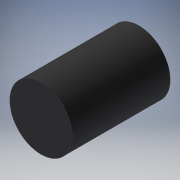
# Autodesk Inventor part: NespressoSpeedfiller-Rod
Saved by Autodesk Inventor 2017 (Build 210142000, 142)
## iProperties
Created: 2018-08-27
Part Number: NespressoSpeedfiller-Rod
Material: Generic
Document SubType Name: Modeling
Designer: 45027374
Density: 1 g/cm^3
Appearance: Default
Author: 45027374
Autodesk Inventor part; units mm, degrees
ref_plane "YZ Plane" through (0, 0, 0) normal (1, 0, 0) x (0, 1, 0)
ref_plane "XZ Plane" through (0, 0, 0) normal (0, 1, 0) x (-1, 0, 0)
ref_plane "XY Plane" through (0, 0, 0) normal (0, 0, 1) x (1, 0, 0)
sketch "Sketch1" plane through (0, 0, 0) normal (0, 1, 0) x (-1, 0, 0)
  line L0 (17.85, 0) -> (-17.85, 0) projected
  line L1 (0, -17.85) -> (0, 17.85) projected
  circle A0 centre (0, 0) radius 12.75
  dimension "d0" = 25.5
  constraints: 1 centre point, 1 coincident
  measures "d0" diameter of A0
extrude "Extrusion1" add sketch "Sketch1" along normal blind 40
body "Solid1"
